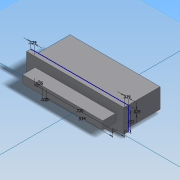
# Autodesk Inventor part: jst-xh 7c
Saved by Autodesk Inventor 2014 SP2 (Build 180246200, 246)
## iProperties
Created: 2014-06-06
Part Number: jst-xh 7c
Material: Generic
Document SubType Name: Modeling
Designer: dliu
Density: 1 g/cm^3
Appearance: Default
Author: dliu
Autodesk Inventor part; units mm, degrees
ref_plane "YZ Plane" through (0, 0, 0) normal (1, 0, 0) x (0, 1, 0)
ref_plane "XZ Plane" through (0, 0, 0) normal (0, 1, 0) x (-1, 0, 0)
ref_plane "XY Plane" through (0, 0, 0) normal (0, 0, 1) x (1, 0, 0)
sketch "Sketch1" plane through (0, 0, 0) normal (0, 0, 1) x (1, 0, 0)
  line L0 (-9.144, 1.9939) -> (9.144, 1.9939)
  line L1 (9.144, 1.9939) -> (9.144, -1.9939)
  line L2 (9.144, -1.9939) -> (-9.144, -1.9939)
  line L3 (-9.144, -1.9939) -> (-9.144, 1.9939)
  line L4 (-9.144, 1.9939) -> (9.144, -1.9939) construction
  line L5 (9.144, 1.9939) -> (-9.144, -1.9939) construction
  line L6 (-9.8806, 2.7305) -> (9.8806, 2.7305)
  line L7 (9.8806, 2.7305) -> (9.8806, -1.9939)
  line L8 (9.8806, -1.9939) -> (-9.8806, -1.9939)
  line L9 (-9.8806, -1.9939) -> (-9.8806, 2.7305)
  line L10 (-7.5438, -1.9939) -> (-6.7818, -1.9939)
  line L11 (-6.7818, -1.9939) -> (-6.7818, -2.8829)
  line L12 (-6.7818, -2.8829) -> (-7.5438, -2.8829)
  line L13 (-7.5438, -2.8829) -> (-7.5438, -1.9939)
  line L14 (-7.5438, -2.8829) -> (7.5438, -2.8829)
  line L15 (7.5438, -2.8829) -> (7.5438, -1.9939)
  line L16 (7.5438, -1.9939) -> (-7.5438, -1.9939)
  line L17 (-7.5438, -1.9939) -> (-7.5438, -2.8829)
  line L18 (7.5438, -1.9939) -> (6.7818, -1.9939)
  line L19 (6.7818, -1.9939) -> (6.7818, -2.8829)
  line L20 (6.7818, -2.8829) -> (7.5438, -2.8829)
  line L21 (7.5438, -2.8829) -> (7.5438, -1.9939)
  line L22 (0, 0) -> (0, -2.8829) construction
  dimension "d0" = 18.288
  dimension "d1" = 3.9878
  dimension "d4" = 0.7366
  dimension "d6" = 0.7366
  dimension "d7" = 0.7366
  dimension "d14" = 0.762
  dimension "d16" = 0.889
  dimension "d17" = 13.5636
  constraints: 46 end point, 10 parallel, 5 horizontal, 5 perpendicular, 3 midpoint, 3 point on line, 2 collinear, 1 coincident, 1 vertical
  measures "d0" distance of L1.end L2.end
  measures "d1" distance of L0.end L1.end
  measures "d4" distance between parallel lines of L0 L6
  measures "d6" distance between parallel lines of L7 L1
  measures "d7" distance between parallel lines of L9 L3
  measures "d14" distance of L11.end L12.end
  measures "d16" distance of L12.end L10.start
  measures "d17" distance between parallel lines of L19 L11
extrude "Extrusion1" add sketch "Sketch1" against normal blind 7.2136 contours L0 L1 L2 L3
extrude "Extrusion2" add sketch "Sketch1" along normal blind 0.8636
sketch "Sketch2" plane through (0, 0, 0.8636) normal (0, 0, 1) x (1, 0, 0)
  line L0 (-8.128, 0.8001) -> (8.128, 0.8001)
  line L1 (8.128, 0.8001) -> (8.128, -0.8001)
  line L2 (8.128, -0.8001) -> (-8.128, -0.8001)
  line L3 (-8.128, -0.8001) -> (-8.128, 0.8001)
  line L4 (8.128, 0.8001) -> (-8.128, -0.8001) construction
  point P0 (0, 0)
  point P1 (0, 0)
  dimension "d10" = 16.256
  dimension "d11" = 1.6002
  constraints: 10 end point, 2 parallel, 1 coincident, 1 horizontal, 1 midpoint, 1 perpendicular
  measures "d10" distance of L1.end L2.end
  measures "d11" distance of L0.end L1.end
extrude "Extrusion3" add sketch "Sketch2" along normal blind 2.54
extrude "Extrusion4" add sketch "Sketch1" against normal blind 5.5372 contours L2 L11 L12 L13 | L15 L14 L19 L2
body "Solid1"
